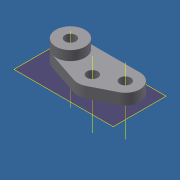
# Autodesk Inventor part: FingerTip_Mount dual
Saved by Autodesk Inventor 2014 SP2 (Build 180246200, 246)
## iProperties
Created: 2014-12-22
Part Number: FingerTip_Mount dual
Material: Generisch
Document SubType Name: Modeling
Designer: 4ndreas
Density: 1 g/cm^3
Appearance: Vorgabe
Mass: 0.495562 g
Surface Area: 6.93822 cm^2
Volume: 0.495562 cm^3
Author: 4ndreas
Autodesk Inventor part; units mm, degrees
ref_plane "YZ Plane" through (0, 0, 0) normal (1, 0, 0) x (0, 1, 0)
ref_plane "XZ Plane" through (0, 0, 0) normal (0, 1, 0) x (-1, 0, 0)
ref_plane "XY Plane" through (0, 0, 0) normal (0, 0, 1) x (1, 0, 0)
sketch "Skizze1" plane through (0, 0, 0) normal (0, 0, 1) x (1, 0, 0)
  line L0 (0, 0) -> (15, 0) construction
  line L1 (9, 0) -> (9, -3) construction
  arc A0 (0, 4) -> (-1.2649, -3.7947) centre (0, 0) ccw
  arc A1 (7.7351, -6.7947) -> (10.7889, -6.5777) centre (9, -3) ccw
  arc A2 (16.7889, -3.5777) -> (15, 4) centre (15, 0) ccw
  line L2 (0, 4) -> (15, 4)
  line L3 (16.7889, -3.5777) -> (10.7889, -6.5777)
  line L4 (7.7351, -6.7947) -> (-1.2649, -3.7947)
  dimension "d0" = 4
  dimension "d1" = 15
  dimension "d2" = 3
  dimension "d6" = 9
  constraints: 10 end point, 6 point on circle, 6 tangent, 3 centre point, 3 coincident, 1 equal radius, 1 horizontal, 1 parallel, 1 perpendicular, 1 point on line
  measures "d0" radius of A0
  measures "d1" distance of L0.start L0.end
  measures "d2" distance of L1.start L1.end
  measures "d6" distance from line of L0.start L1
ref_plane "Arbeitsebene1" through (0, 0, 0) normal (0, 0, -1) x (1, 0, 0)
extrude "Extrusion1" add sketch "Skizze1" along normal blind 3
sketch "Skizze2" plane through (0, 0, 3) normal (0, 0, 1) x (1, 0, 0)
  arc A0 (0, 4) -> (-1.2649, -3.7947) centre (0, 0) ccw projected
  arc A1 (7.7351, -6.7947) -> (10.7889, -6.5777) centre (9, -3) ccw projected
  arc A2 (16.7889, -3.5777) -> (15, 4) centre (15, 0) ccw projected
hole "Bohrung1" at (9, -3, 3) at (15, 0, 3) at (0, 0, 3) direction (0, 0, -1) diameter 3 end through all
sketch "Skizze3" plane through (0, 0, 3) normal (0, 0, 1) x (1, 0, 0)
  circle A0 centre (0, 0) radius 1.5 projected
  arc A1 (0, 4) -> (-1.2649, -3.7947) centre (0, 0) ccw projected
  circle A2 centre (0, 0) radius 4
  constraints: 1 centre point, 1 coincident, 1 concentric
extrude "Extrusion2" add sketch "Skizze3" along normal blind 2.6
equation "\"d0\" = bearingWall"
equation "\"d1\" = Hebel_basis_2"
equation "\"d6\" = 0.6 * d1"
equation "\"d4\" = Join_width"
equation "\"d7\" = bearingHole"
equation "\"FingerLaenge_B\" = 25"
equation "\"Hebel_B\" = 25"
equation "\"Finger_width\" = 22"
equation "\"Finger_diameter\" = 8"
equation "\"FingerWall\" = 3"
equation "\"Hebel_basis_2\" = 15"
equation "\"Join_width\" = 3"
equation "\"bearingHole\" = 3"
equation "\"bearingWall\" = 4"
equation "\"support_D\" = 0.25"
